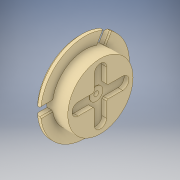
# Autodesk Inventor part: Mouth-Turn-Disk
Saved by Autodesk Inventor 2018.3 (Build 223284000, 284)
## iProperties
Created: 2018-05-19
Part Number: Mouth-Turn-Disk
Material: Generisch
Document SubType Name: Modeling
Designer: JochenAlt
Density: 1 g/cm^3
Appearance: Vorgabe
Author: JochenAlt
Autodesk Inventor part; units mm, degrees
ref_plane "YZ Plane" through (0, 0, 0) normal (1, 0, 0) x (0, 1, 0)
ref_plane "XZ Plane" through (0, 0, 0) normal (0, 1, 0) x (-1, 0, 0)
ref_plane "XY Plane" through (0, 0, 0) normal (0, 0, 1) x (1, 0, 0)
sketch "Skizze1" plane through (0, 0, 0) normal (1, 0, 0) x (0, 1, 0)
  line L0 (0, 19.6) -> (0, -19.6) construction
  line L1 (-19.6, 0) -> (19.6, 0) construction
  circle A0 centre (0, 0) radius 4.15
  arc A1 (2.65, 9.55) -> (-2.65, 9.55) centre (0, 9.55) ccw
  arc A2 (-2.65, -9.55) -> (2.65, -9.55) centre (0, -9.55) ccw
  arc A3 (9.55, -2.65) -> (9.55, 2.65) centre (9.55, 0) ccw
  arc A4 (-9.55, 2.65) -> (-9.55, -2.65) centre (-9.55, 0) ccw
  line L2 (9.55, 2.65) -> (3.1937, 2.65)
  line L3 (-3.1937, 2.65) -> (-9.55, 2.65)
  line L4 (2.65, -9.55) -> (2.65, -3.1937)
  line L5 (2.65, 3.1937) -> (2.65, 9.55)
  line L6 (-2.65, 9.55) -> (-2.65, 3.1937)
  line L7 (-2.65, -3.1937) -> (-2.65, -9.55)
  line L8 (-9.55, -2.65) -> (-3.1937, -2.65)
  line L9 (3.1937, -2.65) -> (9.55, -2.65)
  circle A5 centre (0, 0) radius 14
  circle A6 centre (0, 0) radius 1
  circle A7 centre (0, 0) radius 2.85
  dimension "d0" = 8.3
  dimension "d4" = 24.4
  dimension "d5" = 5.3
  dimension "d6" = 28
  dimension "d14" = 2
  dimension "d15" = 5.7
  constraints: 16 end point, 9 tangent, 8 parallel, 8 point on circle, 7 centre point, 5 equal length, 4 coincident, 4 point on line, 2 horizontal, 2 symmetric about line, 1 equal radius, 10 other
  measures "d5" distance between parallel lines of L7 L4
  measures "d6" diameter of A5
  measures "d14" diameter of A6
  measures "d15" diameter of A7
extrude "Extrusion3" add sketch "Skizze1" along normal blind 4.3 contours A0 | A0 L2 A3 L9 | A0 L6 A1 L5 | L4 A2 L7 A0 | A0 L8 A4 L3 | A5 | A7
extrude "Extrusion1" add sketch "Skizze1" along normal blind 2 from surface at 4.3 contours A5
extrude "Extrusion4" add sketch "Skizze1" along normal blind 0.2 from surface at 4.3 contours A7
extrude "Extrusion7" add sketch "Skizze1" against normal blind 0.3 contours A0 | A0 L2 A3 L9 | A0 L6 A1 L5 | L4 A2 L7 A0 | A0 L8 A4 L3 | A5 | A7
sketch "Skizze3" plane through (0, 0, 0) normal (-1, 0, 0) x (0, 0, 1)
  line L0 (-33.893, 0) -> (33.893, 0) construction
  circle A0 centre (0, 0) radius 15 construction
  line L1 (0, 27.3863) -> (0, -31.318) construction
  line L2 (-1.75, -13.8902) -> (-1.75, -18.9192)
  line L3 (1.75, -18.9192) -> (1.75, -13.8902)
  circle A1 centre (0, 0) radius 4 construction
  line L4 (0, 0) -> (12.9904, 7.5) construction
  line L5 (0, 0) -> (-12.9904, 7.5) construction
  arc A2 (-1.75, -13.8902) -> (1.75, -13.8902) centre (0, 0) ccw
  line L6 (17.2595, 7.9441) -> (12.9043, 5.4296)
  line L7 (15.5095, 10.9752) -> (11.1543, 8.4606)
  arc A3 (12.9043, 5.4296) -> (11.1543, 8.4606) centre (0, 0) ccw
  line L8 (-15.5095, 10.9752) -> (-11.1543, 8.4606)
  line L9 (-17.2595, 7.9441) -> (-12.9043, 5.4296)
  arc A4 (-11.1543, 8.4606) -> (-12.9043, 5.4296) centre (0, 0) ccw
  circle A5 centre (0, 0) radius 14 construction
  arc A6 (1.75, -18.9192) -> (17.2595, 7.9441) centre (0, 0) ccw
  arc A7 (-17.2595, 7.9441) -> (-1.75, -18.9192) centre (0, 0) ccw
  arc A8 (15.5095, 10.9752) -> (-15.5095, 10.9752) centre (0, 0) ccw
  circle A9 centre (0, 0) radius 19 construction
  circle A10 centre (0, 0) radius 4
  point P0 (0, -15)
  dimension "d20" = 30
  dimension "d22" = 3.5
  dimension "d25" = 120
  dimension "d26" = 3.5
  dimension "d27" = 3.5
  dimension "d28" = 38
  constraints: 18 point on circle, 16 end point, 10 centre point, 6 coincident, 3 concentric, 3 parallel, 1 point on line, 6 other
  measures "d20" diameter of A0
  measures "d22" distance between parallel lines of L2 L3
  measures "d25" angle of L5 L4
  measures "d26" distance between parallel lines of L6 L7
  measures "d27" distance between parallel lines of L9 L8
  measures "d28" diameter of A9
extrude "Extrusion6" add sketch "Skizze3" along normal blind 2.4 from surface at 0.3
chamfer "Fase1" distance 1 angle 45 1 edges at (-2.7, 0, -4)
chamfer "Fase2" distance 1 angle 45 3 edges at (-2.7, -9.5, -16.4545) (-2.7, 19, 0) (-2.7, -9.5, 16.4545)
chamfer "Fase3" distance 0.5 angle 45 6 edges at (-0.3, -16.4047, 1.75) (-0.3, -16.4047, -1.75) (-0.3, 6.6868, 15.0819) (-0.3, 9.7179, 13.3319) (-0.3, 9.7179, -13.3319) (-0.3, 6.6868, -15.0819)
equation "\"d26\" = d22"
equation "\"d27\" = d22"
equation "\"d3\" = d2"
equation "\"d2\" = 5"
